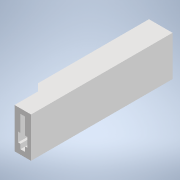
# Autodesk Inventor part: funnel
Saved by Autodesk Inventor 2020 (Build 240168000, 168)
## iProperties
Created: 2019-05-08
Part Number: funnel
Material: Generic
Document SubType Name: Modeling
Designer: erwin
Density: 1 g/cm^3
Appearance: Default
Author: erwin
Autodesk Inventor part; units mm, degrees
ref_plane "YZ Plane" through (0, 0, 0) normal (1, 0, 0) x (0, 1, 0)
ref_plane "XZ Plane" through (0, 0, 0) normal (0, 1, 0) x (-1, 0, 0)
ref_plane "XY Plane" through (0, 0, 0) normal (0, 0, 1) x (1, 0, 0)
sketch "Sketch1" plane through (0, 0, 0) normal (0, 0, 1) x (1, 0, 0)
  arc A0 (16, 5) -> (14, 7) centre (14, 5) ccw projected
  line L0 (14, 7) -> (8, 7) projected
  arc A1 (6, 9) -> (8, 7) centre (8, 9) ccw projected
  line L1 (6, 9) -> (6, 25.5) projected
  arc A2 (6, 25.5) -> (4, 27.5) centre (4, 25.5) ccw projected
  line L2 (4, 27.5) -> (-14, 27.5) projected
  arc A3 (-14, 27.5) -> (-16, 25.5) centre (-14, 25.5) ccw projected
  line L3 (-16, 25.5) -> (-16, 20.5) projected
  line L4 (-16, 20.5) -> (4, 20.5) projected
  line L5 (4, 20.5) -> (4, 5) projected
  line L6 (4, 5) -> (14, 5) projected
  line L7 (14, 5) -> (14, -15) projected
  line L8 (14, -15) -> (4, -15) projected
  line L9 (4, -15) -> (4, -20.5) projected
  line L10 (4, -20.5) -> (-16, -20.5) projected
  line L11 (-16, -20.5) -> (-16, -25.5) projected
  arc A4 (-16, -25.5) -> (-14, -27.5) centre (-14, -25.5) ccw projected
  line L12 (-14, -27.5) -> (4, -27.5) projected
  arc A5 (4, -27.5) -> (6, -25.5) centre (4, -25.5) ccw projected
  line L13 (6, -25.5) -> (6, -19) projected
  arc A6 (8, -17) -> (6, -19) centre (8, -19) ccw projected
  line L14 (8, -17) -> (14, -17) projected
  arc A7 (14, -17) -> (16, -15) centre (14, -15) ccw projected
  line L15 (16, -15) -> (16, 5) projected
  circle A8 centre (-10.2273, -23.9687) radius 0.75 projected
  circle A9 centre (-0.7, 24) radius 0.75 projected
  circle A10 centre (-10.2, 24) radius 0.75 projected
  circle A11 centre (-0.7, -24) radius 0.75 projected
  line L16 (11.5, 0) -> (9.5, 0)
  line L17 (9.5, -13) -> (11.5, -13)
  line L18 (12.5, -11) -> (12.5, -7)
  line L19 (8.5, -7) -> (8.5, -11)
  line L20 (8.5, -11) -> (12.5, -7) construction
  line L21 (12.5, -11) -> (8.5, -7) construction
  line L22 (8.5, -11) -> (9.5, -11)
  line L23 (11.5, -11) -> (12.5, -11)
  line L24 (12.5, -7) -> (11.5, -7)
  line L25 (9.5, -7) -> (8.5, -7)
  line L26 (11.5, -13) -> (11.5, -11)
  line L27 (11.5, -7) -> (11.5, 0)
  line L28 (9.5, 0) -> (9.5, -7)
  line L29 (9.5, -11) -> (9.5, -13)
  line L30 (14, -15) -> (4, -15)
  line L31 (4, -15) -> (4, 2)
  line L32 (4, 2) -> (14, 2)
  line L33 (14, 2) -> (14, -15)
  point P0 (0, 0)
  point P1 (10.5, -9)
  dimension "d0" = 2
  dimension "d1" = 13
  dimension "d2" = 4
  dimension "d3" = 4
  dimension "d5" = 17
  dimension "d6" = 1.5
  dimension "d7" = 2
  dimension "d8" = 2
  dimension "d12" = 1
  dimension "d13" = 1
  constraints: 36 end point, 12 parallel, 5 perpendicular, 4 horizontal, 2 collinear, 2 midpoint
  measures "d0" distance of L17.end L17.start
  measures "d1" distance of L17.start L16.end
  measures "d2" distance of L19.start L18.end
  measures "d3" distance of L18.end L18.start
  measures "d5" distance of L30.end L31.end
  measures "d6" distance between parallel lines of L7 L18
  measures "d7" distance between parallel lines of L32 L16
  measures "d8" distance between parallel lines of L17 L23
  measures "d12" distance of L23.start L18.start
  measures "d13" distance of L19.end L22.end
extrude "Extrusion1" add sketch "Sketch1" along normal blind 50 contours L31 L32 L7 L8
sketch "Sketch2" plane through (0, 0, 50) normal (0, 0, 1) x (1, 0, 0)
  line L0 (14, -15) -> (14, 2) projected
  line L1 (14, 2) -> (4, 2) projected
  line L2 (4, 2) -> (4, -15) projected
  line L3 (4, -15) -> (14, -15) projected
  line L4 (8.5, -7) -> (9.5, -7) projected
  line L5 (9.5, -7) -> (9.5, 0) projected
  line L6 (9.5, 0) -> (11.5, 0) projected
  line L7 (11.5, 0) -> (11.5, -7) projected
  line L8 (11.5, -7) -> (12.5, -7) projected
  line L9 (12.5, -7) -> (12.5, -11) projected
  line L10 (12.5, -11) -> (11.5, -11) projected
  line L11 (11.5, -11) -> (11.5, -13) projected
  line L12 (11.5, -13) -> (9.5, -13) projected
  line L13 (9.5, -13) -> (9.5, -11) projected
  line L14 (9.5, -11) -> (8.5, -11) projected
  line L15 (8.5, -11) -> (8.5, -7) projected
  line L16 (14, 2) -> (4, 2) projected
  line L17 (14, -15) -> (7, -15)
  line L18 (7, -15) -> (7, 2)
  line L19 (7, 2) -> (14, 2)
  line L20 (14, 2) -> (14, -15)
  point P0 (0, 0)
  point P1 (7, 2)
  dimension "d11" = 3
  constraints: 8 end point, 2 parallel, 1 horizontal, 1 perpendicular, 1 point on line
  measures "d11" distance between parallel lines of L2 L18
extrude "Extrusion2" add sketch "Sketch2" along normal blind 10 contours L3 L18 L1 L0
chamfer "Chamfer1" distance 3 angle 45 1 edges at (4, -6.5, 50)
thicken "Thicken1" operation add thickness 0.2 both sides no extend neighbours yes toward (1, 0, 0) faces at (4, -3.6667, 15.6667) (7.3333, -15, 15.6667) (7.3333, 2, 15.6667) (14, -9.3333, 20)
equation "\"d13\" = d12"
body "Solid1"
